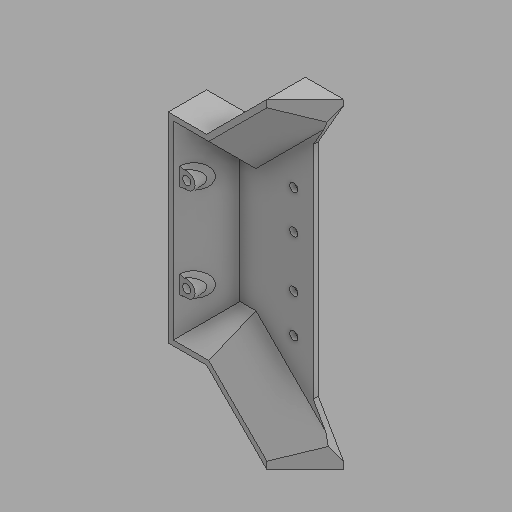
# Autodesk Inventor part: Бампер_задний
Saved by Autodesk Inventor 2025 (Build 290162000, 162)
## iProperties
Created: 2025-04-24
Part Number: Бампер_задний
Material: Типовые
Document SubType Name: Modeling
Designer: Artem Sannikov
Density: 1 g/cm^3
Appearance: По умолчанию
Author: Artem Sannikov
Autodesk Inventor part; units mm, degrees
ref_plane "YZ Plane" through (0, 0, 0) normal (1, 0, 0) x (0, 1, 0)
ref_plane "XZ Plane" through (0, 0, 0) normal (0, 1, 0) x (-1, 0, 0)
ref_plane "XY Plane" through (0, 0, 0) normal (0, 0, 1) x (1, 0, 0)
sketch "Эскиз1" plane through (0, 0, 0) normal (0, 0, 1) x (1, 0, 0)
  line L0 (26.5, 243) -> (73.5, 290) projected
  line L1 (-3.5, 243) -> (26.5, 243) projected
  line L2 (-3.5, 87) -> (26.5, 87) projected
  line L3 (26.5, 87) -> (73.5, 40) projected
  line L4 (-3.5, 340) -> (-3.5, -10) projected
  line L5 (83.5, 340) -> (83.5, -10) projected
  line L6 (103.5, 290) -> (73.5, 290) projected
  line L7 (103.5, 40) -> (73.5, 40) projected
  point P0 (0, 0)
  point P1 (83.5, 40)
  point P2 (83.5, 290)
extrude "Выдавливание1" add sketch "Эскиз1" along normal blind 4
sketch "Эскиз2" plane through (0, 0, 4) normal (0, 0, 1) x (1, 0, 0)
  line L0 (83.5, 40) -> (83.5, 290) projected
  line L1 (26.5, 243) -> (-3.5, 243) projected
  line L2 (-3.5, 243) -> (-3.5, 87) projected
  line L3 (-3.5, 87) -> (26.5, 87) projected
  line L4 (26.5, 87) -> (73.5, 40) projected
  line L5 (73.5, 40) -> (83.5, 40) projected
  line L6 (83.5, 40) -> (83.5, 290) projected
  line L7 (83.5, 290) -> (73.5, 290) projected
  line L8 (73.5, 290) -> (26.5, 243) projected
  line L9 (74.1569, 45) -> (28.1569, 91)
  line L10 (28.1569, 91) -> (0.5, 91)
  line L11 (0.5, 91) -> (0.5, 239)
  line L12 (0.5, 239) -> (28.1569, 239)
  line L13 (28.1569, 239) -> (75.1569, 286)
  line L14 (75.1569, 286) -> (78.5, 286)
  line L15 (78.5, 45) -> (74.1569, 45)
  line L16 (78.5, 286) -> (83.5, 286)
  line L17 (78.5, 45) -> (83.5, 45)
  point P0 (0, 0)
  dimension "d2" = 4
  constraints: 18 end point, 2 point on line, 1 horizontal, 1 perpendicular, 5 other
  measures "d2" distance between parallel lines of L4 L9
extrude "Выдавливание2" add sketch "Эскиз2" along normal up to surface (26 mm away) contours L5 L4 L3 L2 L1 L8 L7 L0 L16 L14 L13 L12 L11 L10 L9 L15 L17
sketch "Эскиз3" plane through (73.5, 290, 0) normal (0, 1, 0) x (1, 0, 0)
  line L0 (30, 0) -> (0, -30) projected
  line L1 (0, -30) -> (30, -30)
  line L2 (30, -30) -> (30, 0)
  point P0 (-73.5, 0)
  constraints: 4 end point, 1 horizontal, 1 perpendicular
extrude "Выдавливание3" cut sketch "Эскиз3" against normal blind 433.5
sketch "Эскиз4" plane through (75.1569, 286, 4) normal (0, -1, 0) x (1, 0, 0)
  line L0 (8.3431, -4) -> (8.3431, 16) projected
  line L1 (28.3431, -4) -> (8.3431, 16)
  line L2 (8.3431, 16) -> (8.3431, -4)
  line L3 (8.3431, -4) -> (28.3431, -4)
  point P0 (-75.1569, -4)
  constraints: 6 end point, 1 collinear, 1 perpendicular, 1 other
extrude "Выдавливание4" add sketch "Эскиз4" against normal up to surface (4 mm away)
sketch "Эскиз5" plane through (74.1569, 45, 4) normal (0, 1, 0) x (1, 0, 0)
  line L0 (9.3431, 4) -> (29.3431, 4) projected
  line L1 (29.3431, 4) -> (9.3431, 4)
  line L2 (9.3431, 4) -> (9.3431, -16)
  line L3 (29.3431, 4) -> (1, -24.3431) projected
  line L4 (9.3431, -16) -> (29.3431, 4)
  point P0 (-74.1569, 4)
  point P1 (9.3431, -16)
  constraints: 6 end point, 1 collinear, 1 horizontal, 1 perpendicular
extrude "Выдавливание5" add sketch "Эскиз5" against normal up to surface (5 mm away)
sketch "Эскиз6" plane through (0, 0, 4) normal (0, 0, 1) x (1, 0, 0)
  line L0 (103.5, 286) -> (103.5, 290) projected
  line L1 (103.5, 286) -> (83.5, 251.359)
  line L2 (83.5, 45) -> (83.5, 286) projected
  line L3 (83.5, 286) -> (103.5, 286)
  line L4 (74.1569, 45) -> (103.5, 45) projected
  line L5 (83.5, 45) -> (103.5, 45)
  line L6 (103.5, 45) -> (83.5, 79.641)
  line L7 (83.5, 79.641) -> (83.5, 45)
  point P0 (0, 0)
  point P1 (74.5, 45)
  dimension "d14" = 30
  dimension "d15" = 30
  constraints: 10 end point, 2 point on line, 1 collinear, 1 perpendicular, 1 vertical
  measures "d14" angle of L1 L2
  measures "d15" angle of L6 L2
extrude "Выдавливание6" add sketch "Эскиз6" against normal up to surface (4 mm away)
sketch "Эскиз7" plane through (73.5, 40, 0) normal (0, -1, 0) x (1, 0, 0)
  line L0 (0.6569, 29.3431) -> (26, 4) projected
  line L1 (23.5208, 6.4792) -> (30.4178, -0.4178)
  line L2 (30.4178, -0.4178) -> (31.9094, 7.9707)
  line L3 (31.9094, 7.9707) -> (23.5208, 6.4792)
  point P0 (-73.5, 0)
  point P1 (26, 4)
  point P2 (26, 4)
  point P3 (1, 30)
  point P4 (10, 21)
  constraints: 6 end point, 3 other
extrude "Выдавливание7" cut sketch "Эскиз7" against normal through all
chamfer "Фаска3" distance 26 angle 45 5 edges at (51.1569, 68, 4) (14.3284, 91, 4) (0.5, 165, 4) (14.3284, 239, 4) (51.6569, 262.5, 4)
chamfer "Фаска4" [suppressed]
sketch "Эскиз8" plane through (0, 0, 4) normal (0, 0, 1) x (1, 0, 0)
  line L0 (78.5, 340) -> (78.5, -10) construction
  line L1 (68.5, 340) -> (68.5, -10) construction
  circle A0 centre (68.5, 215) radius 3.25
  line L2 (68.5, 165) -> (-9.5262, 165) construction
  circle A1 centre (68.5, 185) radius 3.25
  circle A2 centre (68.5, 115) radius 3.25
  circle A3 centre (68.5, 145) radius 3.25
  point P0 (0, 0)
  dimension "d29" = 10
  dimension "d30" = 6.5
  dimension "d31" = 6.5
  dimension "d32" = 20
  dimension "d33" = 30
  constraints: 4 centre point, 4 end point, 2 point on line, 2 symmetric about line, 1 horizontal, 1 midpoint, 1 parallel, 2 other
  measures "d29" distance between parallel lines of L0 L1
  measures "d30" diameter of A0
  measures "d31" diameter of A1
  measures "d32" distance from line of A1.centre L2
  measures "d33" distance of A0.centre A1.centre
extrude "Выдавливание8" cut sketch "Эскиз8" against normal through all
sketch "Эскиз9" plane through (0, 0, 4) normal (0, 0, 1) x (1, 0, 0)
  line L0 (18.5, -10) -> (18.5, 340) construction
  line L1 (8.5, -10) -> (8.5, 340) construction
  line L2 (8.5, 165) -> (33.1999, 165) construction
  circle A0 centre (8.5, 201.5138) radius 6.5
  circle A1 centre (8.5, 128.4862) radius 6.5
  point P0 (0, 0)
  dimension "d36" = 10
  dimension "d37" = 13
  constraints: 4 end point, 2 centre point, 1 horizontal, 1 midpoint, 1 parallel, 1 point on line, 1 symmetric about line, 1 other
  measures "d36" distance between parallel lines of L0 L1
  measures "d37" diameter of A0
extrude "Выдавливание9" add sketch "Эскиз9" along normal blind 23.5
chamfer "Фаска5" distance 2.75 angle 45 4 edges at (10.3028, 207.7588, 20.1972) (10.3028, 195.2688, 20.1972) (10.3028, 134.7312, 20.1972) (10.3028, 122.2412, 20.1972)
sketch "Эскиз10" plane through (0, 0, 27.5) normal (0, 0, 1) x (1, 0, 0)
  arc A0 (6.7261, 122.2329) -> (6.7261, 134.7394) centre (8.5, 128.4862) ccw projected
  arc A1 (6.7261, 195.2606) -> (6.7261, 207.7671) centre (8.5, 201.5138) ccw projected
  circle A2 centre (8.5, 201.5138) radius 3.25
  circle A3 centre (8.5, 128.4862) radius 3.25
  point P0 (0, 0)
  dimension "d43" = 6.5
  dimension "d44" = 6.5
  constraints: 2 centre point, 2 coincident
  measures "d43" diameter of A2
  measures "d44" diameter of A3
extrude "Выдавливание10" cut sketch "Эскиз10" against normal through all
